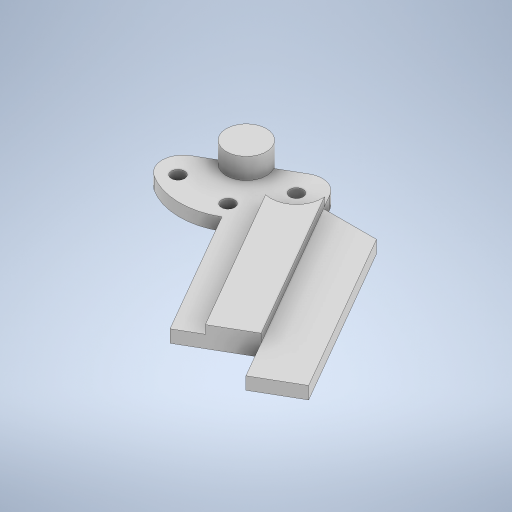
# Autodesk Inventor part: leg_springjoint_bace
Saved by Autodesk Inventor 2024.1 (Build 281209000, 209)
## iProperties
Created: 2024-02-13
Part Number: leg_springjoint_bace
Material: 一般
Document SubType Name: Modeling
Designer: hibik
Density: 1 g/cm^3
Appearance: 既定
Author: hibik
Autodesk Inventor part; units mm, degrees
ref_plane "YZ Plane" through (0, 0, 0) normal (1, 0, 0) x (0, 1, 0)
ref_plane "XZ Plane" through (0, 0, 0) normal (0, 1, 0) x (-1, 0, 0)
ref_plane "XY Plane" through (0, 0, 0) normal (0, 0, 1) x (1, 0, 0)
sketch "スケッチ1" plane through (0, 0, 0) normal (0, 1, 0) x (-1, 0, 0)
  circle A0 centre (0, 0) radius 8
  circle A1 centre (0, 0) radius 6 construction
  circle A2 centre (0, 0) radius 2.4
  circle A3 centre (6, 0) radius 0.8
  circle A4 centre (3, 5.1962) radius 0.8
  circle A5 centre (-3, 5.1962) radius 0.8
  circle A6 centre (-6, 0) radius 0.8
  circle A7 centre (-3, -5.1962) radius 0.8
  circle A8 centre (3, -5.1962) radius 0.8
  line L0 (-6.9282, -4) -> (6.9282, 4)
  line L1 (14.9383, 0) -> (-33.6296, 0) projected
  line L2 (-6.9282, -4) -> (-19.4282, 17.6506)
  line L3 (0, 0) -> (-12.5, 21.6506)
  line L4 (-12.5, 21.6506) -> (-19.4282, 17.6506)
  line L5 (0, 0) -> (-11.6913, -6.75)
  line L6 (-11.6913, -6.75) -> (-26.6913, 19.2308)
  line L7 (-26.6913, 19.2308) -> (-15, 25.9808)
  line L8 (-15, 25.9808) -> (0, 0)
  line L9 (-19.4282, 17.6506) -> (-21.9282, 21.9808)
  point P0 (2.0785, 1.2)
  point P1 (-2.0785, -1.2)
  point P2 (-4, 6.9282)
  point P3 (-15.5885, 0)
  point P4 (-9.2376, 0)
  dimension "d1" = 12
  dimension "d0" = 16
  dimension "d2" = 4.8
  dimension "d3" = 1.6
  dimension "d6" = 360
  dimension "d12" = 30
  dimension "d13" = 25
  dimension "d19" = 13.5
  dimension "d20" = 30
  constraints: 18 end point, 8 centre point, 4 perpendicular, 3 coincident, 2 horizontal alignment, 2 parallel, 2 point on circle, 2 point on line, 1 collinear, 1 midpoint, 15 other
  measures "d0" diameter of A0
  measures "d2" diameter of A2
  measures "d3" diameter of A3
  measures "d12" angle of L1 L0
  measures "d13" distance between parallel lines of L0 L4
  measures "d19" distance between parallel lines of L6 L8
  measures "d20" distance between parallel lines of L7 L5
extrude "押し出し1" add sketch "スケッチ1" along normal blind 1.5 contours L0 A2 L3 A5 A0 | L2 L1 A0 | A0 L1 A6 A2 L0 | L3 A5 A2 L1 A6 A0 | A0 L1 L2 L4 L3 | L1 L6 L7 L9 L2
extrude "押し出し2" add sketch "スケッチ1" along normal blind 4 contours L0 L3 A2 | A2 L1 L0 | L0 L1 A2 | A2 L1 L0 | L3 L1 A2
fillet "フィレット1" radius 2.5 2 edges at (6.9282, 0.75, -4) (-6.9282, 0.75, 4)
sketch "スケッチ2" plane through (0, 1.5, 0) normal (0, 1, 0) x (1, 0, 0)
  point P0 (0, 0)
sketch "スケッチ3" plane through (0, 1.5, 0) normal (0, 1, 0) x (1, 0, 0)
  circle A0 centre (0, 0) radius 2.4 projected
  line L0 (2.0785, 1.2) -> (14.5785, -20.4506)
  line L1 (12.5, -21.6506) -> (19.4282, -17.6506) projected
  line L2 (19.4282, -17.6506) -> (8.1782, 1.8349) projected
  circle A1 centre (0, 0) radius 2.4 projected
  line L3 (15.1847, -20.1006) -> (2.5173, 1.8398)
  arc A2 (8.1782, 1.8349) -> (4.7631, 2.75) centre (6.0131, 0.5849) ccw projected
  line L4 (4.7631, 2.75) -> (2.0785, 1.2) projected
  circle A3 centre (6, 0) radius 3.0851
  circle A4 centre (6, 0) radius 0.8 projected
  point P0 (-1.3153, 8.4782)
  point P1 (10.9282, -2.9282)
  point P2 (4, -6.9282)
  point P3 (2.6847, 1.55)
  point P4 (9.0717, 0.2874)
  point P5 (5.3165, -3.0084)
  point P6 (6.0693, 3.0843)
  point P7 (3.8769, 2.2383)
  point P8 (4.2302, -2.527)
  dimension "d21" = 0.7
  constraints: 4 end point, 4 point on line, 2 parallel, 1 centre point, 1 concentric, 1 tangent, 4 other
  measures "d21" distance between parallel lines of L3 L0
extrude "押し出し3" add sketch "スケッチ3" along normal blind 1 contours A3 L2 L1 L3
